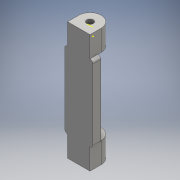
# Autodesk Inventor part: tracks_center_ver2
Saved by Autodesk Inventor 2016 (Build 200138000, 138)
## iProperties
Created: 2016-11-27
Part Number: tracks_center_ver2
Material: Generic
Document SubType Name: Modeling
Designer: hesaon
Density: 1 g/cm^3
Appearance: Default
Author: hesaon
Autodesk Inventor part; units mm, degrees
ref_plane "YZ Plane" through (0, 0, 0) normal (1, 0, 0) x (0, 1, 0)
ref_plane "XZ Plane" through (0, 0, 0) normal (0, 1, 0) x (-1, 0, 0)
ref_plane "XY Plane" through (0, 0, 0) normal (0, 0, 1) x (1, 0, 0)
sketch "Sketch1" plane through (0, 0, 0) normal (0, 1, 0) x (-1, 0, 0)
  line L0 (0, 0) -> (1.1, 0)
  line L1 (1.1, 0) -> (1.1, -2)
  line L2 (1.1, -2) -> (9.6, -2)
  line L3 (9.6, -2) -> (9.6, 0)
  line L4 (9.6, 0) -> (10.7, 0)
  line L5 (10.7, 0) -> (10.7, -29)
  line L6 (10.7, -29) -> (9.6, -29)
  line L7 (9.6, -29) -> (9.6, -27)
  line L8 (9.6, -27) -> (1.1, -27)
  line L9 (1.1, -27) -> (1.1, -29)
  line L10 (1.1, -29) -> (0, -29)
  line L11 (0, -29) -> (0, 0)
  dimension "d7" = 8.5
  dimension "d8" = 8.5
  dimension "d9" = 2
  dimension "d10" = 2
  dimension "d11" = 10.7
  dimension "d12" = 1.1
  dimension "d13" = 1.1
  dimension "d14" = 29
  constraints: 24 end point, 8 perpendicular, 4 point on line, 2 horizontal
  measures "d7" distance of L1.end L2.end
  measures "d8" distance of L8.end L7.end
  measures "d9" distance of L1.end L0.end
  measures "d10" distance of L9.end L8.end
  measures "d11" distance of L0.start L4.end
  measures "d12" distance of L0.start L0.end
  measures "d13" distance of L10.end L9.end
  measures "d14" distance of L10.end L0.start
extrude "Extrusion1" add sketch "Sketch1" along normal blind 4.25
sketch "Sketch4" plane through (-9.6, 0, -2) normal (0, 0, 1) x (1, 0, 0)
  line L0 (8.5, 4.25) -> (0, 4.25) projected
  line L1 (8.5, 4.25) -> (9.6, 4.25) projected
  arc A0 (8.5, 4.25) -> (0, 4.25) centre (4.25, 4.25) ccw
  point P0 (9.6, 0)
  constraints: 2 end point, 2 point on circle, 1 centre point, 1 midpoint
extrude "Extrusion2" add sketch "Sketch4" along normal blind 10
sketch "Sketch5" plane through (-9.6, 0, -2) normal (0, 0, 1) x (1, 0, 0)
  line L0 (0, 0) -> (8.5, 0) projected
  line L1 (9.6, 4.25) -> (8.5, 4.25) projected
  line L2 (0, 0) -> (8.5, 0)
  line L3 (8.5, 0) -> (8.5, 4.25)
  line L4 (8.5, 4.25) -> (0, 4.25)
  line L5 (0, 4.25) -> (0, 0)
  point P0 (9.6, 0)
  constraints: 8 end point, 2 parallel, 1 horizontal, 1 perpendicular
extrude "Extrusion3" add sketch "Sketch5" along normal blind 10
sketch "Sketch6" plane through (-9.6, 0, 8) normal (0, 0, 1) x (1, 0, 0)
  arc A0 (8.5, 4.25) -> (0, 4.25) centre (4.25, 4.25) ccw projected
  circle A1 centre (4.25, 4.25) radius 1.25
  point P0 (9.6, 0)
  dimension "d24" = 2.5
  constraints: 1 centre point, 1 coincident
  measures "d24" diameter of A1
extrude "Extrusion4" cut sketch "Sketch6" against normal blind 10
sketch "Sketch9" plane through (-1.1, 0, -27) normal (0, 0, -1) x (-1, 0, 0)
  line L0 (0, 4.25) -> (8.5, 4.25) projected
  arc A0 (8.5, 4.25) -> (0, 4.25) centre (4.25, 4.25) ccw
  point P0 (-1.1, 0)
  constraints: 2 end point, 2 point on circle, 1 centre point, 1 midpoint
extrude "Extrusion6" add sketch "Sketch9" along normal blind 10
sketch "Sketch10" plane through (-1.1, 0, -27) normal (0, 0, -1) x (-1, 0, 0)
  line L0 (8.5, 4.25) -> (9.6, 4.25) projected
  line L1 (0, 0) -> (8.5, 0)
  line L2 (8.5, 0) -> (8.5, 4.25)
  line L3 (8.5, 4.25) -> (0, 4.25)
  line L4 (0, 4.25) -> (0, 0)
  point P0 (-1.1, 0)
  constraints: 8 end point, 2 parallel, 1 horizontal, 1 perpendicular
extrude "Extrusion7" add sketch "Sketch10" along normal blind 10
sketch "Sketch11" plane through (-1.1, 0, -37) normal (0, 0, -1) x (-1, 0, 0)
  arc A0 (5.5, 4.25) -> (3, 4.25) centre (4.25, 4.25) ccw projected
  line L0 (8.5, 4.25) -> (5.5, 4.25) projected
  circle A1 centre (4.25, 4.25) radius 1.25
  point P0 (-1.1, 0)
  constraints: 1 coincident, 1 horizontal alignment, 2 other
extrude "Extrusion8" cut sketch "Sketch11" against normal blind 10
sketch "Sketch13" plane through (0, 4.25, 0) normal (0, 1, 0) x (1, 0, 0)
  line L0 (0, 29) -> (0, 0) projected
  line L1 (0, 0) -> (0, 29)
  line L2 (-1.1, 29) -> (0, 29) projected
  line L3 (0, 29) -> (-1.1, 29)
  line L4 (-1.1, 29) -> (-1.1, 27) projected
  line L5 (-1.1, 29) -> (-1.1, 27)
  line L6 (-6.6, 27) -> (-9.6, 27) projected
  line L7 (-1.1, 27) -> (-9.6, 27)
  line L8 (-9.6, 27) -> (-9.6, 29) projected
  line L9 (-9.6, 27) -> (-9.6, 29)
  line L10 (-10.7, 29) -> (-9.6, 29) projected
  line L11 (-9.6, 29) -> (-10.7, 29)
  line L12 (-10.7, 0) -> (-10.7, 29) projected
  line L13 (-10.7, 29) -> (-10.7, 0)
  line L14 (-9.6, 0) -> (-9.6, 2) projected
  line L15 (-10.7, 0) -> (-9.6, 0)
  line L16 (-9.6, 0) -> (-9.6, 2)
  line L17 (-4.1, 2) -> (-1.1, 2) projected
  line L18 (-9.6, 2) -> (-1.1, 2)
  line L19 (0, 0) -> (-1.1, 0) projected
  line L20 (-1.1, 2) -> (-1.1, 0)
  line L21 (-1.1, 0) -> (0, 0)
  constraints: 24 end point, 6 collinear, 6 perpendicular
extrude "Extrusion9" cut sketch "Sketch13" against normal blind 1.25
chamfer "Chamfer1" distance 2 angle 45 3 edges at (-5.35, 8.5, -2) (-1.1, 3.625, -2) (-9.6, 3.625, -2)
chamfer "Chamfer2" distance 2 angle 45 3 edges at (-5.35, 8.5, -27) (-1.1, 3.625, -27) (-9.6, 3.625, -27)
fillet "Fillet1" radius 1.1 4 edges at (0, 1.5, 0) (0, 1.5, -29) (-10.7, 1.5, 0) (-10.7, 1.5, -29)
sketch "Sketch14" plane through (-9.6, 0, 8) normal (0, 0, 1) x (1, 0, 0)
  line L0 (4.25, 3) -> (6.5, 3) projected
  point P0 (9.6, 0)
body "Solid1"
